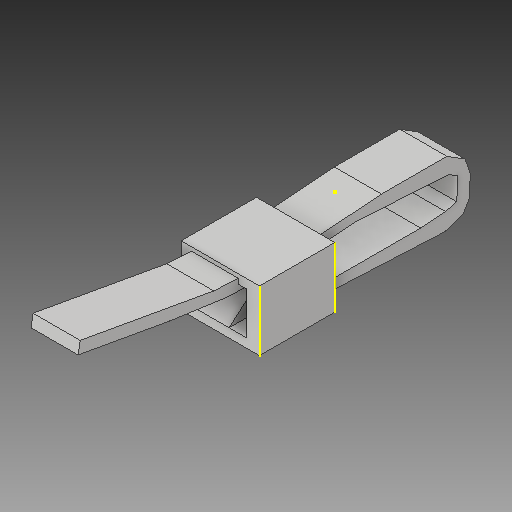
# Autodesk Inventor part: Ziptie
Saved by Autodesk Inventor 2018 (Build 220112000, 112)
## iProperties
Created: 2016-08-11
Part Number: Ziptie
Material: Generic
Document SubType Name: Modeling
Designer: User
Density: 1 g/cm^3
Appearance: Default
Author: User
Autodesk Inventor part; units mm, degrees
ref_plane "YZ Plane" through (0, 0, 0) normal (1, 0, 0) x (0, 1, 0)
ref_plane "XZ Plane" through (0, 0, 0) normal (0, 1, 0) x (-1, 0, 0)
ref_plane "XY Plane" through (0, 0, 0) normal (0, 0, 1) x (1, 0, 0)
sketch "Sketch1" plane through (0, 0, 0) normal (0, 0, 1) x (1, 0, 0)
  line L0 (92.558, -5.5266) -> (88.4016, -5.5266)
  line L1 (88.4016, -5.5266) -> (88.4016, -2.3241)
  line L2 (88.4016, -2.3241) -> (92.558, -2.3241)
  line L3 (92.558, -2.3241) -> (92.558, -5.5266)
  line L4 (91.8766, -5.0496) -> (88.9467, -5.0496)
  line L5 (88.9467, -5.0496) -> (88.9467, -2.8011)
  line L6 (88.9467, -2.8011) -> (91.8766, -2.8011)
  line L7 (91.8766, -2.8011) -> (91.8766, -5.0496)
  point P0 (0, 0)
  constraints: 16 end point, 4 parallel, 2 horizontal, 2 perpendicular
extrude "Extrusion1" add sketch "Sketch1" along normal blind 4
sketch "Sketch3" plane through (92.558, -5.5266, 0) normal (1, 0, 0) x (0, 0, -1)
  line L0 (-4, 0) -> (-4, 3.2025) projected
  line L1 (0, 3.2025) -> (0, 0) projected
  point P0 (0, 5.5266)
sketch "Sketch4" plane through (88.9467, -5.0496, 0) normal (1, 0, 0) x (0, 0, -1)
  line L0 (0, 2.7255) -> (0, -0.477) projected
  line L1 (0, -0.477) -> (4.8951, -0.7122)
  line L2 (4.8951, -0.7122) -> (7.0077, -0.8137)
  line L3 (7.0077, -0.8137) -> (7.9085, -0.5009)
  line L4 (7.9085, -0.5009) -> (8.2533, 0.0718)
  line L5 (8.2533, 0.0718) -> (8.3068, 1.1847)
  line L6 (8.3068, 1.1847) -> (8.0262, 1.993)
  line L7 (8.0262, 1.993) -> (7.0621, 2.6005)
  line L8 (7.0621, 2.6005) -> (3.5876, 2.6005)
  line L9 (3.5876, 2.6005) -> (-0.3844, 2.3008)
  line L10 (-0.3844, 2.3008) -> (-5.3135, 2.6005)
  line L11 (-5.3135, 2.6005) -> (-8.9119, 3.2451)
  line L12 (-8.9119, 3.2451) -> (-12.4072, 3.8713)
  line L13 (-12.4072, 3.8713) -> (-12.517, 3.2581)
  line L14 (-12.517, 3.2581) -> (-7.6517, 2.3865)
  line L15 (-7.6517, 2.3865) -> (-4.6985, 1.9752)
  line L16 (-4.6985, 1.9752) -> (-0.7689, 1.7864)
  line L17 (-0.7689, 1.7864) -> (2.2504, 2.0142)
  line L18 (2.2504, 2.0142) -> (6.5148, 1.7549)
  line L19 (6.5148, 1.7549) -> (7.1634, 1.7155)
  line L20 (7.1634, 1.7155) -> (7.6433, 1.4131)
  line L21 (7.6433, 1.4131) -> (7.6418, 1.3822)
  line L22 (7.6418, 1.3822) -> (7.5978, 0.465)
  line L23 (7.5978, 0.465) -> (7.5874, 0.25)
  line L24 (7.5874, 0.25) -> (6.9873, 0.0994)
  line L25 (6.9873, 0.0994) -> (5.6698, 0)
  line L26 (0, 0) -> (-4, 0) projected
  line L27 (5.6698, 0) -> (0, 0)
  line L28 (0, 0) -> (0, -0.477)
  point P0 (0, 5.0496)
  constraints: 54 end point, 10 point on line, 7 parallel, 5 perpendicular
extrude "Extrusion2" add sketch "Sketch4" along normal blind 2.5 contours L27 L25 L24 L23 L22 L21 L20 L19 L18 L17 L0 L9 L8 L7 L6 L5 L4 L3 L2 L1 | L17 L16 L15 L14 L13 L12 L11 L10 L9 L0
sketch "Sketch5" plane through (88.9467, -5.0496, 4) normal (1, 0, 0) x (0, 0, -1)
  line L0 (4, 0) -> (0, 0) projected
  line L1 (0, 0) -> (0.9929, 0)
  line L2 (0.9929, 0) -> (1.9546, 1.1114)
  line L3 (1.9546, 1.1114) -> (1.4737, 1.2793)
  line L4 (0, 0) -> (0, 1.9416) projected
  line L5 (1.4737, 1.2793) -> (0, 0)
  point P0 (4, 5.0496)
  constraints: 8 end point, 1 point on line
extrude "Extrusion3" add sketch "Sketch5" along normal blind 2
body "Solid1"
